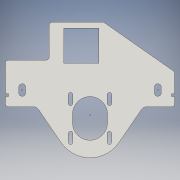
# Autodesk Inventor part: Gantry Outer
Saved by Autodesk Inventor 2018.2 (Build 222227000, 227)
## iProperties
Created: 2017-12-19
Part Number: Gantry Outer
Material: Steel
Document SubType Name: Modeling
Designer: torba
Density: 7.85 g/cm^3
Appearance: Steel
Author: torba
Autodesk Inventor part; units mm, degrees
ref_plane "YZ Plane" through (0, 0, 0) normal (1, 0, 0) x (0, 1, 0)
ref_plane "XZ Plane" through (0, 0, 0) normal (0, 1, 0) x (-1, 0, 0)
ref_plane "XY Plane" through (0, 0, 0) normal (0, 0, 1) x (1, 0, 0)
sketch "Sketch1" plane through (0, 0, 0) normal (0, 1, 0) x (-1, 0, 0)
  line L0 (19.05, 0) -> (203.2, 0)
  line L1 (203.2, 0) -> (203.2, -368.3)
  line L2 (203.2, -368.3) -> (19.05, -368.3)
  line L3 (19.05, -368.3) -> (19.05, 0)
  line L4 (190.5, -127) -> (113.792, -127)
  line L5 (113.792, -127) -> (113.792, -203.708)
  line L6 (113.792, -203.708) -> (190.5, -203.708)
  line L7 (190.5, -203.708) -> (190.5, -127)
  line L8 (203.2, -95.25) -> (120.65, -95.25)
  line L9 (120.65, -95.25) -> (120.65, 0)
  line L10 (203.2, -196.85) -> (203.2, -215.9)
  line L11 (120.65, -95.25) -> (120.65, -368.3) construction
  line L12 (19.05, 0) -> (19.05, -184.15)
  line L13 (19.05, 0) -> (38.1, 0)
  line L14 (38.1, 0) -> (38.1, -368.3) construction
  line L15 (38.1, -368.3) -> (19.05, -368.3)
  line L16 (19.05, -368.3) -> (19.05, 0)
  line L17 (38.1, -368.3) -> (38.1, -331.75) construction
  line L18 (38.1, 0) -> (38.1, -36.55) construction
  line L19 (38.1, -36.55) -> (55.6, -36.55) construction
  line L20 (38.1, -331.75) -> (55.6, -331.75) construction
  circle A0 centre (55.6, -36.55) radius 17.5 construction
  circle A1 centre (55.6, -331.75) radius 17.5 construction
  line L21 (19.05, -147.6) -> (19.05, -122.2)
  line L22 (19.05, -233.4) -> (19.05, -258.8)
  circle A2 centre (55.6, -331.75) radius 7.5
  circle A3 centre (55.6, -36.55) radius 7.5
  line L23 (19.05, 0) -> (19.05, -132.5921)
  line L24 (19.05, -368.3) -> (19.05, -248.4079)
  line L25 (19.05, -368.3) -> (95.25, -368.3)
  line L26 (19.05, -265.1125) -> (19.05, -115.8875)
  line L27 (19.05, -55.772) -> (19.05, -155.2732)
  line L28 (19.05, -227.7309) -> (19.05, -312.528)
  line L29 (203.2, -184.15) -> (203.2, -213.868)
  line L30 (203.2, -213.868) -> (95.25, -368.3)
  line L31 (95.25, -368.3) -> (203.2, -368.3)
  line L32 (203.2, -368.3) -> (203.2, -213.868)
  line L33 (190.5, -203.708) -> (203.2, -203.708)
  point P0 (0, 0)
  point P1 (74.65, -368.3)
  dimension "d0" = 184.15
  dimension "d1" = 368.3
  dimension "d2" = 76.708
  dimension "d3" = 12.7
  dimension "d6" = 31.75
  dimension "d7" = 82.55
  dimension "d8" = 76.708
  dimension "d12" = 19.05
  dimension "d13" = 36.55
  dimension "d14" = 36.55
  dimension "d15" = 17.5
  dimension "d16" = 17.5
  dimension "d19" = 15
  dimension "d20" = 15
  dimension "d30" = 76.2
  dimension "d67" = 95.25
  dimension "d68" = 203.2
  dimension "d69" = 95.25
  dimension "d70" = 101.6
  dimension "d88" = 10.16
  dimension "d89" = 76.708
  dimension "d209" = 34.954
  constraints: 68 end point, 23 point on line, 7 horizontal, 6 parallel, 6 perpendicular, 4 coincident, 3 centre point, 3 collinear, 2 midpoint, 1 horizontal alignment, 1 tangent, 2 other
  measures "d0" distance of L1.end L2.end
  measures "d1" distance of L0.end L1.end
  measures "d2" distance of L6.end L5.end
  measures "d3" distance between parallel lines of L1 L7
  measures "d6" distance between parallel lines of L4 L8
  measures "d7" distance of L8.start L8.end
  measures "d8" distance between parallel lines of L6 L4
  measures "d12" distance of L14.end L15.end
  measures "d13" distance of L14.end L17.end
  measures "d14" distance of L13.end L18.end
  measures "d15" distance of L18.end L19.end
  measures "d16" distance of L17.end L20.end
  measures "d19" diameter of A2
  measures "d20" diameter of A3
  measures "d30" distance of L15.end L25.end
  measures "d67" distance between parallel lines of L0 L8
  measures "d68" distance from line of point (0, 0) L1
  measures "d69" distance from line of point (0, 0) L8
  measures "d70" distance from line of L10.start L8
  measures "d88" distance from line of L33 L29.end
  measures "d89" distance between parallel lines of L5 L7
  measures "d209" angle of L30 L1
extrude "Extrusion2" add sketch "Sketch1" along normal blind 6.35 contours L0 L9 L8 L1 L30 L2 L3
fillet "Fillet2" radius 6.35 7 edges at (-203.2, 3.175, -95.25) (-120.65, 3.175, -95.25) (-120.65, 3.175, 0) (-19.05, 3.175, 0) (-19.05, 3.175, -368.3) (-95.25, 3.175, -368.3) (-203.2, 3.175, -213.868)
sketch "Sketch4" plane through (0, 6.35, 0) normal (0, 1, 0) x (1, 0, 0)
  line L0 (-19.05, 6.35) -> (-19.05, 361.95) projected
  arc A0 (-19.05, 361.95) -> (-25.4, 368.3) centre (-25.4, 361.95) ccw projected
  line L1 (-25.4, 368.3) -> (-91.9412, 368.3) projected
  arc A1 (-91.9412, 368.3) -> (-97.1457, 365.588) centre (-91.9412, 361.95) ccw projected
  line L2 (-97.1457, 365.588) -> (-202.0545, 215.5067) projected
  arc A2 (-202.0545, 215.5067) -> (-203.2, 211.8687) centre (-196.85, 211.8687) ccw projected
  line L3 (-203.2, 211.8687) -> (-203.2, 101.6) projected
  arc A3 (-203.2, 101.6) -> (-196.85, 95.25) centre (-196.85, 101.6) ccw projected
  line L4 (-196.85, 95.25) -> (-127, 95.25) projected
  arc A4 (-120.65, 88.9) -> (-127, 95.25) centre (-127, 88.9) ccw projected
  line L5 (-120.65, 88.9) -> (-120.65, 6.35) projected
  arc A5 (-120.65, 6.35) -> (-114.3, 0) centre (-114.3, 6.35) ccw projected
  line L6 (-114.3, 0) -> (-25.4, 0) projected
  arc A6 (-25.4, 0) -> (-19.05, 6.35) centre (-25.4, 6.35) ccw projected
  line L7 (-190.5, 127) -> (-190.5, 203.708) projected
  line L8 (-190.5, 203.708) -> (-113.792, 203.708) projected
  line L9 (-113.792, 203.708) -> (-113.792, 127) projected
  line L10 (-113.792, 127) -> (-190.5, 127) projected
  circle A7 centre (-55.6, 36.55) radius 7.5 projected
  circle A8 centre (-55.6, 331.75) radius 7.5 projected
  circle A9 centre (-55.6, 331.75) radius 7.5 projected
  line L11 (-55.6, 331.75) -> (-55.6, 36.55)
  line L12 (-55.6, 184.15) -> (6.249, 184.15) construction
  line L13 (6.249, 184.15) -> (15.774, 184.15) construction
  line L14 (6.249, 184.15) -> (26.95, 184.15) construction
  line L15 (-3.276, 184.15) -> (15.774, 184.15) construction
  line L16 (-3.276, 146.05) -> (15.774, 146.05)
  line L17 (15.774, 222.25) -> (-3.276, 222.25)
  arc A10 (-3.276, 222.25) -> (-3.276, 146.05) centre (-3.276, 184.15) ccw
  arc A11 (15.774, 146.05) -> (15.774, 222.25) centre (15.774, 184.15) ccw
  line L18 (15.774, 184.15) -> (42.7148, 211.0908)
  line L19 (15.774, 184.15) -> (53.874, 184.15) construction
  line L20 (-31.2368, 184.15) -> (94.4868, 184.15) construction
  line L21 (53.874, 184.15) -> (79.274, 184.15)
  line L22 (-19.05, 6.35) -> (-19.05, 361.95) projected
  line L23 (-19.05, 68.099) -> (58.745, 121.222)
  line L24 (-19.05, 300.201) -> (58.745, 247.078)
  arc A12 (58.745, 121.222) -> (58.745, 247.078) centre (15.774, 184.15) ccw
  point P0 (0, 0)
  point P1 (95.125, 171.45)
  dimension "d101" = 61.849
  dimension "d102" = 9.525
  dimension "d104" = 76.2
  dimension "d109" = 45
  dimension "d112" = 25.4
  dimension "d126" = 114.175
  dimension "d127" = 171.45
  dimension "d128" = 113.5368
  dimension "d129" = 12.1868
  dimension "d145" = 76.2
  dimension "d146" = 55.672
  dimension "d147" = 55.672
  dimension "d148" = 19.05
  constraints: 28 end point, 7 point on circle, 6 tangent, 5 point on line, 3 centre point, 3 horizontal, 2 collinear, 2 midpoint, 1 coincident, 1 equal length, 1 parallel, 1 vertical
  measures "d101" distance of L12.start L12.end
  measures "d102" distance of L12.end L13.end
  measures "d104" diameter of A11
  measures "d109" angle of L19 L18
  measures "d112" distance of L19.end L21.end
  measures "d126" distance from line of point (95.125, 171.45) L22
  measures "d127" distance from line of point (95.125, 171.45) L6
  measures "d128" distance from line of L20.end L22
  measures "d129" distance from line of L20.start L22
  measures "d145" radius of A12
  measures "d146" angle of L22 L24
  measures "d147" angle of L23 L0
  measures "d148" distance of L16.start L16.end
extrude "Extrusion8" add sketch "Sketch4" against normal up to surface (6.35 mm away) contours A6 L6 A5 L5 A4 L4 A3 L3 A2 L2 A1 L1 A0 L0 A10 | L0 A10 L16 A11 L17 L24 A12 L23 | A10 L0 | L0 A10 L17 A11 L16 | L7 L8 L9 L10 | A7 | A8
extrude "Extrusion9" cut sketch "Sketch4" against normal blind 25.4 contours A10 L0 | L0 A10 L17 A11 L16
extrude "Extrusion10" cut sketch "Sketch1" along normal blind 25.4 contours L7 L6 L5 L4 | A2 | A3
fillet "Fillet6" radius 12.7 2 edges at (-19.05, 3.175, -68.099) (-19.05, 3.175, -300.201)
sketch "Sketch5" plane through (0, 6.35, 0) normal (0, 1, 0) x (1, 0, 0)
  circle A0 centre (-55.6, 36.55) radius 7.5 projected
  circle A1 centre (-55.6, 331.75) radius 7.5 projected
  line L0 (-190.5, 203.708) -> (-113.792, 203.708) projected
  line L1 (-113.792, 203.708) -> (-113.792, 127) projected
  line L2 (-113.792, 127) -> (-190.5, 127) projected
  line L3 (-190.5, 127) -> (-190.5, 203.708) projected
  arc A2 (15.774, 146.05) -> (15.774, 222.25) centre (15.774, 184.15) ccw projected
  line L4 (15.774, 146.05) -> (-3.276, 146.05) projected
  arc A3 (-3.276, 222.25) -> (-3.276, 146.05) centre (-3.276, 184.15) ccw projected
  line L5 (-3.276, 222.25) -> (15.774, 222.25) projected
  arc A4 (-202.0545, 215.5067) -> (-203.2, 211.8687) centre (-196.85, 211.8687) ccw projected
  line L6 (-203.2, 211.8687) -> (-203.2, 101.6) projected
  arc A5 (-203.2, 101.6) -> (-196.85, 95.25) centre (-196.85, 101.6) ccw projected
  line L7 (-196.85, 95.25) -> (-127, 95.25) projected
  arc A6 (-120.65, 88.9) -> (-127, 95.25) centre (-127, 88.9) ccw projected
  line L8 (-120.65, 88.9) -> (-120.65, 6.35) projected
  arc A7 (-120.65, 6.35) -> (-114.3, 0) centre (-114.3, 6.35) ccw projected
  line L9 (-114.3, 0) -> (-25.4, 0) projected
  arc A8 (-25.4, 0) -> (-19.05, 6.35) centre (-25.4, 6.35) ccw projected
  line L10 (-19.05, 6.35) -> (-19.05, 61.3928) projected
  arc A9 (-13.5118, 71.8808) -> (-19.05, 61.3928) centre (-6.35, 61.3928) ccw projected
  line L11 (-13.5118, 71.8808) -> (58.745, 121.222) projected
  arc A10 (58.745, 121.222) -> (58.745, 247.078) centre (15.774, 184.15) ccw projected
  line L12 (58.745, 247.078) -> (-13.5118, 296.4192) projected
  arc A11 (-19.05, 306.9072) -> (-13.5118, 296.4192) centre (-6.35, 306.9072) ccw projected
  line L13 (-19.05, 306.9072) -> (-19.05, 361.95) projected
  arc A12 (-19.05, 361.95) -> (-25.4, 368.3) centre (-25.4, 361.95) ccw projected
  line L14 (-25.4, 368.3) -> (-91.9412, 368.3) projected
  arc A13 (-91.9412, 368.3) -> (-97.1457, 365.588) centre (-91.9412, 361.95) ccw projected
  line L15 (-97.1457, 365.588) -> (-202.0545, 215.5067) projected
  line L16 (-49.25, 36.55) -> (-61.95, 36.55) construction
  line L17 (-49.25, 44.05) -> (-61.95, 44.05)
  line L18 (-61.95, 29.05) -> (-49.25, 29.05)
  arc A14 (-49.25, 29.05) -> (-49.25, 44.05) centre (-49.25, 36.55) ccw
  arc A15 (-61.95, 44.05) -> (-61.95, 29.05) centre (-61.95, 36.55) ccw
  line L19 (-49.25, 331.75) -> (-61.95, 331.75) construction
  line L20 (-49.25, 339.25) -> (-61.95, 339.25)
  line L21 (-61.95, 324.25) -> (-49.25, 324.25)
  arc A16 (-49.25, 324.25) -> (-49.25, 339.25) centre (-49.25, 331.75) ccw
  arc A17 (-61.95, 339.25) -> (-61.95, 324.25) centre (-61.95, 331.75) ccw
  point P0 (0, 0)
  dimension "d133" = 6.35
  dimension "d134" = 15
  dimension "d135" = 6.35
  dimension "d136" = 15
  constraints: 16 end point, 8 point on circle, 8 tangent, 4 centre point, 3 parallel, 2 midpoint, 1 horizontal
  measures "d133" distance of A0.centre L16.end
  measures "d134" diameter of A15
  measures "d135" distance of A1.centre L19.end
  measures "d136" diameter of A17
extrude "Extrusion11" cut sketch "Sketch5" against normal blind 25.4 contours A0 L17 A14 L18 | A0 L18 A15 L17 | A1 L20 A16 L21 | A1 L21 A17 L20
sketch "Sketch8" plane through (0, 6.35, 0) normal (0, 1, 0) x (1, 0, 0)
  line L0 (-61.95, 44.05) -> (-49.25, 44.05) projected
  arc A0 (-49.25, 29.05) -> (-49.25, 44.05) centre (-49.25, 36.55) ccw projected
  line L1 (-49.25, 29.05) -> (-61.95, 29.05) projected
  arc A1 (-61.95, 44.05) -> (-61.95, 29.05) centre (-61.95, 36.55) ccw projected
  line L2 (-61.95, 339.25) -> (-49.25, 339.25) projected
  arc A2 (-49.25, 324.25) -> (-49.25, 339.25) centre (-49.25, 331.75) ccw projected
  line L3 (-49.25, 324.25) -> (-61.95, 324.25) projected
  arc A3 (-61.95, 339.25) -> (-61.95, 324.25) centre (-61.95, 331.75) ccw projected
  line L4 (-190.5, 203.708) -> (-113.792, 203.708) projected
  line L5 (-113.792, 203.708) -> (-113.792, 127) projected
  line L6 (-113.792, 127) -> (-190.5, 127) projected
  line L7 (-190.5, 127) -> (-190.5, 203.708) projected
  arc A4 (15.774, 146.05) -> (15.774, 222.25) centre (15.774, 184.15) ccw projected
  line L8 (15.774, 146.05) -> (-3.276, 146.05) projected
  arc A5 (-3.276, 222.25) -> (-3.276, 146.05) centre (-3.276, 184.15) ccw projected
  line L9 (-3.276, 222.25) -> (15.774, 222.25) projected
  arc A6 (-202.0545, 215.5067) -> (-203.2, 211.8687) centre (-196.85, 211.8687) ccw projected
  line L10 (-203.2, 211.8687) -> (-203.2, 101.6) projected
  arc A7 (-203.2, 101.6) -> (-196.85, 95.25) centre (-196.85, 101.6) ccw projected
  line L11 (-196.85, 95.25) -> (-127, 95.25) projected
  arc A8 (-120.65, 88.9) -> (-127, 95.25) centre (-127, 88.9) ccw projected
  line L12 (-120.65, 88.9) -> (-120.65, 6.35) projected
  arc A9 (-120.65, 6.35) -> (-114.3, 0) centre (-114.3, 6.35) ccw projected
  line L13 (-114.3, 0) -> (-25.4, 0) projected
  arc A10 (-25.4, 0) -> (-19.05, 6.35) centre (-25.4, 6.35) ccw projected
  line L14 (-19.05, 6.35) -> (-19.05, 61.3928) projected
  arc A11 (-13.5118, 71.8808) -> (-19.05, 61.3928) centre (-6.35, 61.3928) ccw projected
  line L15 (-13.5118, 71.8808) -> (58.745, 121.222) projected
  arc A12 (58.745, 121.222) -> (58.745, 247.078) centre (15.774, 184.15) ccw projected
  line L16 (58.745, 247.078) -> (-13.5118, 296.4192) projected
  arc A13 (-19.05, 306.9072) -> (-13.5118, 296.4192) centre (-6.35, 306.9072) ccw projected
  line L17 (-19.05, 306.9072) -> (-19.05, 361.95) projected
  arc A14 (-19.05, 361.95) -> (-25.4, 368.3) centre (-25.4, 361.95) ccw projected
  line L18 (-25.4, 368.3) -> (-91.9412, 368.3) projected
  arc A15 (-91.9412, 368.3) -> (-97.1457, 365.588) centre (-91.9412, 361.95) ccw projected
  line L19 (-97.1457, 365.588) -> (-202.0545, 215.5067) projected
  line L20 (-26.5121, 141.8768) -> (-45.5621, 141.8768) construction
  line L21 (-26.5121, 146.779) -> (-45.5621, 146.779)
  line L22 (-45.5621, 136.9746) -> (-26.5121, 136.9746)
  arc A16 (-26.5121, 136.9746) -> (-26.5121, 146.779) centre (-26.5121, 141.8768) ccw
  arc A17 (-45.5621, 146.779) -> (-45.5621, 136.9746) centre (-45.5621, 141.8768) ccw
  line L23 (-26.4992, 226.431) -> (-45.5492, 226.431) construction
  line L24 (-26.4992, 231.3332) -> (-45.5492, 231.3332)
  line L25 (-45.5492, 221.5288) -> (-26.4992, 221.5288)
  arc A18 (-26.4992, 221.5288) -> (-26.4992, 231.3332) centre (-26.4992, 226.431) ccw
  arc A19 (-45.5492, 231.3332) -> (-45.5492, 221.5288) centre (-45.5492, 226.431) ccw
  line L26 (58.0601, 226.4232) -> (39.0101, 226.431) construction
  line L27 (58.0621, 231.3254) -> (39.0121, 231.3332)
  line L28 (39.0081, 221.5288) -> (58.0581, 221.521)
  arc A20 (58.0581, 221.521) -> (58.0621, 231.3254) centre (58.0601, 226.4232) ccw
  arc A21 (39.0121, 231.3332) -> (39.0081, 221.5288) centre (39.0101, 226.431) ccw
  line L29 (58.0517, 141.8639) -> (39.0017, 141.8768) construction
  line L30 (58.055, 146.7661) -> (39.005, 146.779)
  line L31 (38.9983, 136.9746) -> (58.0483, 136.9617)
  arc A22 (58.0483, 136.9617) -> (58.055, 146.7661) centre (58.0517, 141.8639) ccw
  arc A23 (39.005, 146.779) -> (38.9983, 136.9746) centre (39.0017, 141.8768) ccw
  point P0 (0, 0)
  point P1 (-36.0371, 141.8768)
  point P2 (-36.0242, 226.431)
  point P3 (48.5351, 226.4271)
  point P4 (48.5267, 141.8703)
  dimension "d191" = 84.5593
  dimension "d192" = 84.5593
  dimension "d193" = 84.5638
  dimension "d194" = 84.5542
  dimension "d195" = 19.05
  dimension "d196" = 9.8044
  dimension "d197" = 19.05
  dimension "d198" = 9.8044
  dimension "d199" = 19.05
  dimension "d200" = 9.8044
  dimension "d201" = 19.05
  dimension "d202" = 9.8044
  dimension "d203" = 34.304
  dimension "d204" = 80.381
  dimension "d205" = 15.7529
  dimension "d206" = 100.3124
  constraints: 32 end point, 16 point on circle, 16 tangent, 8 centre point, 5 parallel, 4 midpoint, 2 point on line, 1 horizontal
  measures "d191" distance of L26.start L29.start
  measures "d192" distance of L23.start L26.start
  measures "d193" distance of L20.start L29.start
  measures "d194" distance of L23.start L20.start
  measures "d195" distance of L20.start L20.end
  measures "d196" diameter of A17
  measures "d197" distance of L23.start L23.end
  measures "d198" diameter of A19
  measures "d199" distance of L26.start L26.end
  measures "d200" diameter of A21
  measures "d201" distance of L29.start L29.end
  measures "d202" diameter of A23
  measures "d203" angle of L16 L27
  measures "d204" distance between parallel lines of L8 L23
  measures "d205" distance from line of L16.start L27
  measures "d206" distance from line of L16.start L30
extrude "Extrusion15" cut sketch "Sketch8" against normal blind 25.4 contours A16 L22 A17 L21 | A18 L25 A19 L24 | A20 L28 A21 L27 | A22 L31 A23 L30
sketch "Sketch10" plane through (0, 6.35, 0) normal (0, 1, 0) x (1, 0, 0)
  line L0 (-49.25, 29.05) -> (-61.95, 29.05) projected
  line L1 (-61.95, 44.05) -> (-49.25, 44.05) projected
  line L2 (-49.25, 324.25) -> (-61.95, 324.25) projected
  line L3 (-61.95, 339.25) -> (-49.25, 339.25) projected
  line L4 (-55.6, 29.05) -> (-55.6, 44.05)
  line L5 (-55.6, 324.25) -> (-55.6, 339.25)
  circle A0 centre (-55.6, 36.55) radius 1.27
  circle A1 centre (-55.6, 331.75) radius 1.27
  point P0 (0, 0)
  dimension "d210" = 2.54
  dimension "d211" = 2.54
  constraints: 6 midpoint, 4 end point, 2 centre point
  measures "d210" diameter of A0
  measures "d211" diameter of A1
extrude "Extrusion16" add sketch "Sketch10" against normal up to surface (6.35 mm away) separate body
sketch "Sketch11" plane through (-25.4, 6.35, -368.3) normal (0, 0, -1) x (-1, 0, 0)
  line L0 (66.5412, 0) -> (66.5412, -6.35) projected
  line L1 (0, 0) -> (66.5412, 0) projected
  line L2 (0, -6.35) -> (0, 0) projected
  line L3 (0, -6.35) -> (66.5412, -6.35) projected
  line L4 (0, 0) -> (66.5412, 0) projected
  line L5 (0, 0) -> (15.875, 0)
  line L6 (0, -6.35) -> (66.5412, -6.35) projected
  line L7 (15.875, 0) -> (22.225, 0)
  line L8 (22.225, 0) -> (22.225, -6.35)
  line L9 (22.225, -6.35) -> (15.875, -6.35)
  line L10 (15.875, -6.35) -> (15.875, 0)
  dimension "d214" = 15.875
  dimension "d215" = 6.35
  constraints: 10 end point, 2 parallel, 2 point on line, 1 horizontal, 1 perpendicular
  measures "d214" distance of L1.start L5.end
  measures "d215" distance of L8.end L9.end
extrude "Extrusion17" cut sketch "Sketch11" against normal blind 6.35 contours L8 L3 L10 L1 bodies 1
sketch "Sketch12" plane through (-114.3, 6.35, 0) normal (0, 0, 1) x (1, 0, 0)
  line L0 (88.9, 0) -> (88.9, -6.35) projected
  line L1 (0, 0) -> (88.9, 0) projected
  line L2 (0, -6.35) -> (0, 0) projected
  line L3 (0, -6.35) -> (88.9, -6.35) projected
  line L4 (66.675, 0) -> (66.675, -6.35) projected
  line L5 (73.025, -6.35) -> (73.025, 0) projected
  point P0 (114.3, -6.35)
extrude "Extrusion18" cut sketch "Sketch12" against normal blind 6.35 contours L5 L3 L4 L1 bodies 1
sketch "Sketch13" plane through (0, 6.35, 0) normal (0, 1, 0) x (1, 0, 0)
  arc A0 (39.0121, 231.3332) -> (39.0081, 221.5288) centre (39.0101, 226.431) ccw construction
  line L0 (39.0121, 231.3332) -> (58.0621, 231.3254) construction
  arc A1 (58.0581, 221.521) -> (58.0621, 231.3254) centre (58.0601, 226.4232) ccw construction
  line L1 (58.0581, 221.521) -> (39.0081, 221.5288) construction
  arc A2 (-45.5621, 146.779) -> (-45.5621, 136.9746) centre (-45.5621, 141.8768) ccw construction
  line L2 (-45.5621, 146.779) -> (-26.5121, 146.779) construction
  arc A3 (-26.5121, 136.9746) -> (-26.5121, 146.779) centre (-26.5121, 141.8768) ccw construction
  line L3 (-26.5121, 136.9746) -> (-45.5621, 136.9746) construction
  arc A4 (-45.5492, 231.3332) -> (-45.5492, 221.5288) centre (-45.5492, 226.431) ccw construction
  line L4 (-45.5492, 231.3332) -> (-26.4992, 231.3332) construction
  arc A5 (-26.4992, 221.5288) -> (-26.4992, 231.3332) centre (-26.4992, 226.431) ccw construction
  line L5 (-26.4992, 221.5288) -> (-45.5492, 221.5288) construction
  arc A6 (39.005, 146.779) -> (38.9983, 136.9746) centre (39.0017, 141.8768) ccw construction
  line L6 (39.005, 146.779) -> (58.055, 146.7661) construction
  arc A7 (58.0483, 136.9617) -> (58.055, 146.7661) centre (58.0517, 141.8639) ccw construction
  line L7 (58.0483, 136.9617) -> (38.9983, 136.9746) construction
  line L8 (-61.95, 44.05) -> (-49.25, 44.05) construction
  arc A8 (-49.25, 29.05) -> (-49.25, 44.05) centre (-49.25, 36.55) ccw construction
  line L9 (-49.25, 29.05) -> (-61.95, 29.05) construction
  arc A9 (-61.95, 44.05) -> (-61.95, 29.05) centre (-61.95, 36.55) ccw construction
  line L10 (-61.95, 339.25) -> (-49.25, 339.25) construction
  arc A10 (-49.25, 324.25) -> (-49.25, 339.25) centre (-49.25, 331.75) ccw construction
  line L11 (-49.25, 324.25) -> (-61.95, 324.25) construction
  arc A11 (-61.95, 339.25) -> (-61.95, 324.25) centre (-61.95, 331.75) ccw construction
  line L12 (-190.5, 203.708) -> (-113.792, 203.708) construction
  line L13 (-113.792, 203.708) -> (-113.792, 127) construction
  line L14 (-113.792, 127) -> (-190.5, 127) construction
  line L15 (-190.5, 127) -> (-190.5, 203.708) construction
  arc A12 (15.774, 146.05) -> (15.774, 222.25) centre (15.774, 184.15) ccw construction
  line L16 (15.774, 146.05) -> (-3.276, 146.05) construction
  arc A13 (-3.276, 222.25) -> (-3.276, 146.05) centre (-3.276, 184.15) ccw construction
  line L17 (-3.276, 222.25) -> (15.774, 222.25) construction
  line L18 (-47.625, 0) -> (-47.625, 6.35) construction
  line L19 (-47.625, 6.35) -> (-41.275, 6.35) construction
  line L20 (-41.275, 6.35) -> (-41.275, 0) construction
  line L21 (-41.275, 0) -> (-25.4, 0) construction
  arc A14 (-25.4, 0) -> (-19.05, 6.35) centre (-25.4, 6.35) ccw construction
  line L22 (-19.05, 6.35) -> (-19.05, 61.3928) construction
  arc A15 (-13.5118, 71.8808) -> (-19.05, 61.3928) centre (-6.35, 61.3928) ccw construction
  line L23 (-13.5118, 71.8808) -> (58.745, 121.222) construction
  arc A16 (58.745, 121.222) -> (58.745, 247.078) centre (15.774, 184.15) ccw construction
  line L24 (58.745, 247.078) -> (-13.5118, 296.4192) construction
  arc A17 (-19.05, 306.9072) -> (-13.5118, 296.4192) centre (-6.35, 306.9072) ccw construction
  line L25 (-19.05, 306.9072) -> (-19.05, 361.95) construction
  arc A18 (-19.05, 361.95) -> (-25.4, 368.3) centre (-25.4, 361.95) ccw construction
  line L26 (-25.4, 368.3) -> (-41.275, 368.3) construction
  line L27 (-41.275, 368.3) -> (-41.275, 361.95) construction
  line L28 (-41.275, 361.95) -> (-47.625, 361.95) construction
  line L29 (-47.625, 361.95) -> (-47.625, 368.3) construction
  line L30 (-47.625, 368.3) -> (-91.9412, 368.3) construction
  arc A19 (-91.9412, 368.3) -> (-97.1457, 365.588) centre (-91.9412, 361.95) ccw construction
  line L31 (-97.1457, 365.588) -> (-202.0545, 215.5067) construction
  arc A20 (-202.0545, 215.5067) -> (-203.2, 211.8687) centre (-196.85, 211.8687) ccw construction
  line L32 (-203.2, 211.8687) -> (-203.2, 101.6) construction
  arc A21 (-203.2, 101.6) -> (-196.85, 95.25) centre (-196.85, 101.6) ccw construction
  line L33 (-196.85, 95.25) -> (-127, 95.25) construction
  arc A22 (-120.65, 88.9) -> (-127, 95.25) centre (-127, 88.9) ccw construction
  line L34 (-120.65, 88.9) -> (-120.65, 6.35) construction
  arc A23 (-120.65, 6.35) -> (-114.3, 0) centre (-114.3, 6.35) ccw construction
  line L35 (-114.3, 0) -> (-47.625, 0) construction
  line L36 (-19.05, 306.9072) -> (-19.05, 361.95) construction
  line L37 (-19.05, 6.35) -> (-19.05, 61.3928) construction
  line L38 (-19.05, 306.9072) -> (-19.05, 61.3928) construction
  line L39 (-19.05, 306.9072) -> (-19.05, 361.95) construction
  line L40 (-19.05, 306.9072) -> (-12.573, 306.9072) construction
  line L41 (-12.573, 306.9072) -> (-12.573, 61.3928) construction
  line L42 (-12.573, 61.3928) -> (-19.05, 61.3928) construction
  line L43 (-19.05, 61.3928) -> (-19.05, 306.9072) construction
  line L44 (-3.276, 184.15) -> (-19.05, 184.15)
  line L45 (-12.573, 184.15) -> (-0.5842, 184.15)
  circle A24 centre (-0.5842, 184.15) radius 1.27
  point P0 (0, 0)
  dimension "d220" = 6.477
  dimension "d221" = 11.9888
  dimension "d222" = 2.54
  constraints: 14 end point, 3 parallel, 2 midpoint, 2 point on line, 1 centre point, 1 coincident, 1 collinear, 1 horizontal, 1 perpendicular
  measures "d220" distance of L41.end L42.end
  measures "d221" distance of L45.start L45.end
  measures "d222" diameter of A24
extrude "Extrusion19" add sketch "Sketch13" against normal blind 6.35 bodies 1
equation "\"d14\" = d13"
equation "\"d16\" = d15"
body "Solid2"
body "Solid3"
